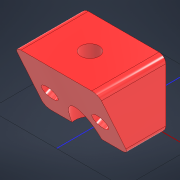
# Autodesk Inventor part: Camera-Mount
Saved by Autodesk Inventor 2022.2 (Build 262287010, 287A)
## iProperties
Created: 2022-04-02
Part Number: Camera-Mount
Material: ABS-Kunststoff
Document SubType Name: Modeling
Designer: sleib
Density: 1.06 g/cm^3
Appearance: Hellrot
Author: sleib
Autodesk Inventor part; units mm, degrees
ref_plane "YZ Plane" through (0, 0, 0) normal (1, 0, 0) x (0, 1, 0)
ref_plane "XZ Plane" through (0, 0, 0) normal (0, 1, 0) x (-1, 0, 0)
sketch "Skizze1" plane through (0, 0, 0) normal (1, 0, 0) x (0, 1, 0)
  line L0 (0, 0) -> (20, 0)
  line L1 (20, 0) -> (20, 20)
  line L2 (20, 20) -> (0, 10.9276)
  line L3 (0, 10.9276) -> (0, 0)
  dimension "d0" = 20
  dimension "d2" = 24.4
  dimension "d18" = 20
  constraints: 8 end point, 1 horizontal, 1 parallel, 1 perpendicular
  measures "d0" distance of L0.start L0.end
  measures "d2" angle of L0 L2
  measures "d18" distance of L0.end L1.end
extrude "Extrusion1" add sketch "Skizze1" along normal mid plane 25
sketch "Skizze2" plane through (-12.5, 0, 10.9276) normal (0, -0.4131, 0.9107) x (1, 0, 0)
  line L0 (0, 0) -> (0, 21.9615) projected
  line L1 (0, 21.9615) -> (25, 21.9615) projected
  line L2 (25, 21.9615) -> (25, 0) projected
  line L3 (25, 0) -> (0, 0) projected
  line L4 (0, 21.9615) -> (25, 21.9615) projected
  line L5 (12.5, 21.9615) -> (12.5, 0) construction
  line L6 (0, 0) -> (25, 0) projected
  circle A0 centre (5, 8.5) radius 2.35
  circle A1 centre (20, 8.5) radius 2.35
  point P0 (12.5, -4.5142)
  dimension "d5" = 4.7
  dimension "d6" = 15
  dimension "d7" = 8.5
  constraints: 2 centre point, 2 end point, 2 midpoint, 1 equal radius, 1 horizontal alignment, 1 symmetric about line
  measures "d5" diameter of A0
  measures "d6" distance of A1.centre A0.centre
  measures "d7" distance from line of L3 A0.centre
extrude "Extrusion2" cut sketch "Skizze2" against normal blind 5 contours A0 | A1
ref_plane "Arbeitsebene3" through (-12.5, 14, 20) normal (0, 1, 0) x (1, 0, 0)
sketch "Skizze5" plane through (-12.5, 14, 20) normal (0, 1, 0) x (1, 0, 0)
  line L0 (0, 0) -> (25, 0) projected
  line L1 (25, 20) -> (25, 0) projected
  line L2 (25, 20) -> (0, 20) projected
  line L3 (0, 0) -> (0, 20) projected
  line L4 (12.5, 0) -> (12.5, 20) construction
  line L5 (0, 10) -> (25, 10) construction
  circle A0 centre (12.5, 10) radius 2.7
  circle A1 centre (12.5, 10) radius 4.5
  dimension "d20" = 5.4
  dimension "d21" = 9
  constraints: 4 end point, 4 midpoint, 2 centre point, 1 coincident, 1 perpendicular
  measures "d20" diameter of A0
  measures "d21" diameter of A1
extrude "Extrusion5" cut sketch "Skizze5" along normal through all contours A0
extrude "Extrusion6" cut sketch "Skizze5" against normal through all contours A0 | A1
fillet "Rundung1" radius 2 4 edges at (12.5, 0, 5.4638) (12.5, 20, 10) (-12.5, 0, 5.4638) (-12.5, 20, 10)
